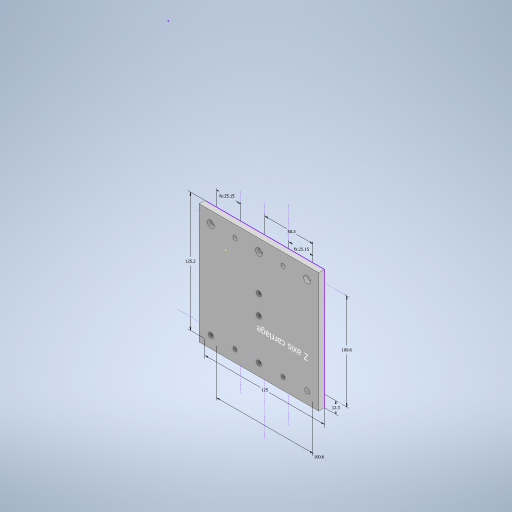
# Autodesk Inventor part: Z axis carriage small
Saved by Autodesk Inventor 2023.2 (Build 272271000, 271)
## iProperties
Created: 2023-05-09
Part Number: Z axis carriage small
Material: Generic
Document SubType Name: Modeling
Designer: dmargari
Density: 1 g/cm^3
Appearance: Default
Author: dmargari
## iProperties of the stored document X axis carriage small_3DPrint.ipt
Created: 2023-05-12
Part Number: X axis carriage small_3DPrint
Material: Generic
Document SubType Name: Modeling
Designer: dmargari
Density: 1 g/cm^3
Appearance: Default
Author: dmargari
Autodesk Inventor part; units mm, degrees
ref_plane "YZ Plane" through (0, 0, 0) normal (1, 0, 0) x (0, 1, 0)
ref_plane "XZ Plane" through (0, 0, 0) normal (0, 1, 0) x (-1, 0, 0)
ref_plane "XY Plane" through (0, 0, 0) normal (0, 0, 1) x (1, 0, 0)
sketch "Sketch1" plane through (0, 0, 0) normal (0, 0, 1) x (1, 0, 0)
  line L0 (97.2346, 27.952) -> (-27.7654, 27.952)
  line L1 (-27.7654, 27.952) -> (-27.7654, -97.248)
  line L2 (-27.7654, -97.248) -> (97.2346, -97.248)
  line L3 (97.2346, -97.248) -> (97.2346, 27.952)
  line L4 (85.1346, 27.952) -> (85.1346, -97.248) construction
  line L5 (-15.4654, 27.952) -> (-15.4654, -97.248) construction
  line L6 (-37.3152, 15.652) -> (117.1466, 15.652) construction
  line L7 (115.2487, -84.948) -> (-56.3615, -84.948) construction
  line L8 (34.8346, -156.7023) -> (34.8346, 57.8793) construction
  line L9 (59.9846, 68.2484) -> (59.9846, -132.2245) construction
  line L10 (9.6846, 55.4717) -> (9.6846, -128.574) construction
  point P0 (0, 0)
  point P1 (-65.7997, 171.2688)
  point P2 (85.1346, -84.948)
  point P3 (85.1346, 15.652)
  point P4 (-15.4654, 15.652)
  point P5 (-15.4654, -84.948)
  point P6 (34.8346, -84.948)
  point P7 (34.8346, 15.652)
  point P8 (59.9846, 15.652)
  point P9 (9.6846, 15.652)
  point P10 (59.9846, -84.948)
  point P11 (9.6846, -84.948)
  dimension "d0" = 125
  dimension "d1" = 125.2
  dimension "d6" = 100.6
  dimension "d48" = 12.3
  dimension "d49" = 100.6
  dimension "d50" = 50.3
  dimension "d72" = 25.15
  dimension "d73" = 25.15
  constraints: 24 point on line, 22 end point, 4 perpendicular, 3 vertical, 2 horizontal, 2 parallel
  measures "d0" distance of L2.end L1.end
  measures "d1" distance of L1.end L0.end
  measures "d6" distance between parallel lines of L4 L5
  measures "d48" distance between parallel lines of L2 L7
  measures "d49" distance between parallel lines of L7 L6
  measures "d50" distance between parallel lines of L4 L8
  measures "d72" distance between parallel lines of L4 L9
  measures "d73" distance between parallel lines of L5 L10
extrude "Extrusion1" add sketch "Sketch1" along normal blind 6
hole "Hole6" at (85.1346, -84.948, 0) at (34.8346, -84.948, 0) at (-15.4654, -84.948, 0) direction (0, 0, 1) diameter 5.1 end through all counterbore diameter 9.2 counterbore depth 2
sketch "Sketch2" plane through (0, 0, 6) normal (0, 0, 1) x (1, 0, 0)
  line L0 (86.1945, -57.9789) -> (32.1694, -57.9789) construction
  line L1 (32.1694, -57.9789) -> (32.1694, -50.1092) construction
  line L2 (32.1694, -50.1092) -> (86.1945, -50.1092) construction
  line L3 (86.1945, -50.1092) -> (86.1945, -57.9789) construction
  point P0 (0, 0)
  constraints: 2 other
sketch "Sketch3" plane through (0, 0, 0) normal (0, 0, -1) x (-1, 0, 0)
  point P0 (0, 0)
hole "Hole7" at (85.1346, 15.652, 0) at (34.8346, 15.652, 0) at (-15.4654, 15.652, 0) direction (0, 0, 1) diameter 7.2 end through all counterbore diameter 12.25 counterbore depth 2
sketch "Sketch5" plane through (0, 0, 0) normal (0, 0, -1) x (-1, 0, 0)
  point P0 (0, 0)
  point P1 (-34.7346, -22.248)
  point P2 (-34.7346, -42.248)
hole "Hole8" at (34.7346, -22.248, 0) at (34.7346, -42.248, 0) direction (0, 0, 1) diameter 5.1 end through all counterbore diameter 9.2 counterbore depth 2
hole "Hole9" at (59.9846, 15.652, 0) at (9.6846, 15.652, 0) at (59.9846, -84.948, 0) at (9.6846, -84.948, 0) direction (0, 0, 1) diameter 4.2 end through all
equation "\"d72\" = 0.5 * d50"
equation "\"d73\" = 0.5 * d50"
body "Solid1"
